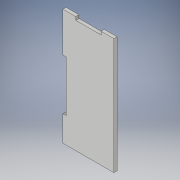
# Autodesk Inventor part: side
Saved by Autodesk Inventor 2017 (Build 210142000, 142)
## iProperties
Created: 2017-06-27
Part Number: side
Material: Generic
Document SubType Name: Modeling
Designer: millerid
Density: 1 g/cm^3
Appearance: Default
Author: millerid
Autodesk Inventor part; units mm, degrees
ref_plane "YZ Plane" through (0, 0, 0) normal (1, 0, 0) x (0, 1, 0)
ref_plane "XZ Plane" through (0, 0, 0) normal (0, 1, 0) x (-1, 0, 0)
ref_plane "XY Plane" through (0, 0, 0) normal (0, 0, 1) x (1, 0, 0)
sketch "Sketch1" plane through (0, 0, 0) normal (0, 0, 1) x (1, 0, 0)
  line L0 (50.8, 115.57) -> (50.8, 0)
  line L1 (50.8, 0) -> (0, 0)
  line L2 (0, 115.57) -> (12.8016, 115.57)
  line L3 (12.8016, 115.57) -> (12.8016, 112.395)
  line L4 (12.8016, 112.395) -> (37.9984, 112.395)
  line L5 (37.9984, 112.395) -> (37.9984, 115.57)
  line L6 (37.9984, 115.57) -> (50.8, 115.57)
  line L7 (0, 0) -> (0, 25.5016)
  line L8 (0, 25.5016) -> (3.175, 25.5016)
  line L9 (3.175, 25.5016) -> (3.175, 76.0984)
  line L10 (3.175, 76.0984) -> (0, 76.0984)
  line L11 (0, 76.0984) -> (0, 115.57)
  dimension "d0" = 115.57
  dimension "d1" = 50.8
  dimension "d2" = 12.8016
  dimension "d3" = 3.175
  dimension "d4" = 25.1968
  dimension "d7" = 25.5016
  dimension "d8" = 3.175
  dimension "d9" = 50.5968
  constraints: 24 end point, 3 perpendicular, 1 horizontal, 1 vertical
  measures "d0" distance of L1.end L2.start
  measures "d1" distance of L2.start L0.start
  measures "d2" distance of L2.start L2.end
  measures "d3" distance of L2.end L3.end
  measures "d4" distance of L3.end L4.end
  measures "d7" distance of L1.end L7.end
  measures "d8" distance of L7.end L8.end
  measures "d9" distance of L8.end L9.end
extrude "Extrusion1" add sketch "Sketch1" along normal blind 3.175
body "Solid1"
